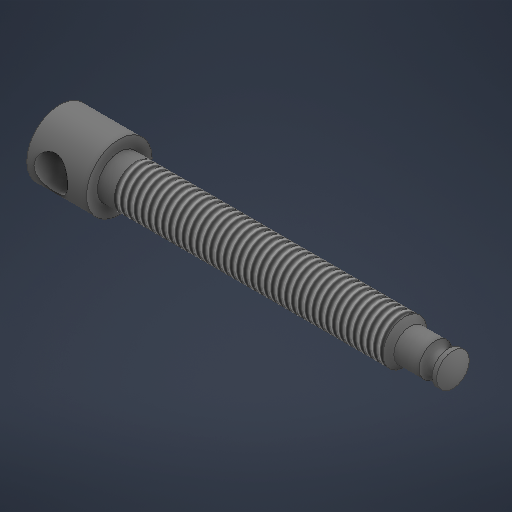
# Autodesk Inventor part: Menetesorsó
Saved by Autodesk Inventor 2025 (Build 290162010, 162A)
## iProperties
Created: 2025-02-13
Part Number: Menetesorsó
Material: Generic
Document SubType Name: Modeling
Designer: petruska.milan
Density: 1 g/cm^3
Appearance: Default
Author: petruska.milan
Autodesk Inventor part; units mm, degrees
ref_plane "YZ Plane" through (0, 0, 0) normal (1, 0, 0) x (0, 1, 0)
ref_plane "XZ Plane" through (0, 0, 0) normal (0, 1, 0) x (-1, 0, 0)
sketch "Sketch1" plane through (0, 0, 0) normal (0, 0, 1) x (1, 0, 0)
  line L0 (0, 0) -> (74, 0)
  line L1 (0, 0) -> (17, 0)
  circle A0 centre (17, 0) radius 17
  line L2 (0, 0) -> (0, 12)
  line L3 (74, 0) -> (69, 0)
  circle A1 centre (69, 0) radius 5
  line L4 (74, 0) -> (74, 3)
  line L5 (74, 3) -> (65.2, 3)
  line L6 (65.2, 3) -> (65.2, 0)
  line L7 (65.2, 0) -> (74, 0)
  line L8 (74, 0) -> (74, 3)
  line L9 (74, 3) -> (69.8, 3)
  line L10 (69.8, 3) -> (69.8, 3)
  line L11 (69.8, 0) -> (74, 0)
  line L12 (74, 0) -> (74, 3)
  line L13 (74, 0) -> (69.8, 0)
  line L14 (69.8, 0) -> (69.8, 1.8)
  line L15 (71, 1.8) -> (74, 1.8)
  line L16 (74, 1.8) -> (74, 0)
  arc A2 (69.8, 3) -> (71, 1.8) centre (71, 3) ccw
  line L17 (71, 1.8) -> (71, 1.8)
  line L18 (72.2, 3) -> (72.2, 3)
  arc A3 (71, 1.8) -> (72.2, 3) centre (71, 3) ccw
  line L19 (65.2, 0) -> (12, 0)
  line L20 (12, 0) -> (12, 4)
  line L21 (12, 4) -> (65.2, 4)
  line L22 (65.2, 4) -> (65.2, 0)
  line L23 (12, 0) -> (0, 0)
  line L24 (0, 0) -> (0, 6)
  line L25 (0, 6) -> (12, 6)
  line L26 (12, 6) -> (12, 0)
  line L27 (12, 6) -> (5.5, 6)
  line L28 (5.5, 6) -> (5.5, 0)
  point P0 (72.2, 1.8)
  point P1 (1.094, 6)
  point P2 (73, 3)
  dimension "d0" = 74
  dimension "d1" = 17
  dimension "d2" = 12
  dimension "d3" = 5
  dimension "d4" = 3
  dimension "d5" = 8.8
  dimension "d6" = 4.2
  dimension "d7" = 1.8
  dimension "d8" = 1.2
  dimension "d9" = 1.2
  dimension "d10" = 1.2
  dimension "d11" = 53.2
  dimension "d12" = 4
  dimension "d13" = 6
  dimension "d14" = 6.5
  constraints: 58 end point, 12 point on line, 10 parallel, 9 perpendicular, 6 horizontal, 4 point on circle, 4 tangent, 2 centre point, 2 coincident, 2 vertical, 1 midpoint, 6 other
  measures "d0" distance of L0.start L0.end
  measures "d1" distance of L0.start L1.end
  measures "d2" distance of L0.start L2.end
  measures "d3" distance of L0.end L3.end
  measures "d4" distance of L0.end L4.end
  measures "d5" distance of L7.end L6.end
  measures "d6" distance of L11.end L11.start
  measures "d7" distance of L14.end L13.end
  measures "d8" radius of A2
  measures "d9" distance of L15.start point (72.2, 1.8)
  measures "d10" radius of A3
  measures "d11" distance of L20.end L21.end
  measures "d12" distance of L19.end L20.end
  measures "d13" distance of L23.end L24.end
  measures "d14" distance of L25.end L27.end
revolve "Revolution1" add sketch "Sketch1" angle 360 about axis through (65.2, 0, 0) along (-1, 0, 0) contours A0 L25 L28 L0 | L28 L25 L26 L20 L0 | A0 L21 L22 A1 L0 | L0 L20 L21 A0 | A1 L22 L6 L0 | L6 L5 A2 L15 A1 L0 | A1 L15 A3 L5
chamfer "Chamfer1" distance 1 angle 45 1 edges at (65.2, -4, 0)
ref_plane "Work Plane1" through (6.547, 0, 6) normal (0, 0, 1) x (1, 0, 0)
sketch "Sketch2" plane through (6.547, 0, 6) normal (0, 0, 1) x (1, 0, 0)
  line L0 (5.453, 4) -> (5.453, -4) projected
  line L1 (5.453, 0) -> (-1.047, 0)
  circle A0 centre (-1.047, 0) radius 3.1
  point P0 (-6.547, 0)
  dimension "d19" = 6.5
  dimension "d20" = 6.2
  constraints: 2 end point, 1 centre point, 1 coincident, 1 horizontal, 1 midpoint
  measures "d19" distance of L1.start L1.end
  measures "d20" diameter of A0
extrude "Extrusion1" cut sketch "Sketch2" against normal through all
thread "Thread1" size "M8x1.25" class "6g" standard "ANSI Metric M Profile" length 49.2
body "Solid1"
